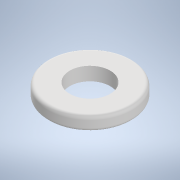
# Autodesk Inventor part: Pieza1
Saved by Autodesk Inventor 2020.3 (Build 243373010, 373A)
## iProperties
Created: 2020-11-12
Part Number: Pieza1
Material: Acero, galvanizado
Document SubType Name: Modeling
Designer: codig
Density: 7.85 g/cm^3
Appearance: Galvanizado
Author: codig
Autodesk Inventor part; units mm, degrees
ref_plane "YZ Plane" through (0, 0, 0) normal (1, 0, 0) x (0, 1, 0)
ref_plane "XZ Plane" through (0, 0, 0) normal (0, 1, 0) x (-1, 0, 0)
ref_plane "XY Plane" through (0, 0, 0) normal (0, 0, 1) x (1, 0, 0)
sketch "Boceto1" plane through (0, 0, 0) normal (0, 1, 0) x (-1, 0, 0)
  circle A0 centre (0, 0) radius 3
  circle A1 centre (0, 0) radius 6.25
  constraints: 2 centre point, 2 coincident
extrude "Extrusión1" add sketch "Boceto1" along normal blind 2
fillet "Empalme1" radius 0.5 1 edges at (6.25, 2, 0)
fillet "Empalme2" radius 0.5 1 edges at (6.25, 0, 0)
